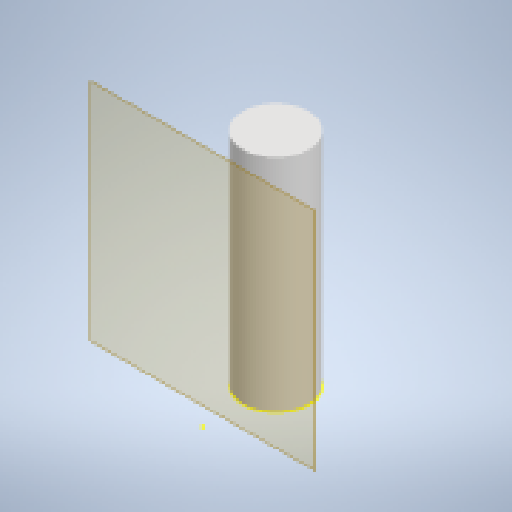
# Autodesk Inventor part: 21700
Saved by Autodesk Inventor 2024.2 (Build 282272000, 272)
## iProperties
Created: 2025-10-05
Part Number: 21700
Material: Типовые
Document SubType Name: Modeling
Designer: katya_notebook
Density: 1 g/cm^3
Appearance: По умолчанию
Author: katya_notebook
Autodesk Inventor part; units mm, degrees
ref_plane "YZ Plane" through (0, 0, 0) normal (1, 0, 0) x (0, 1, 0)
ref_plane "XZ Plane" through (0, 0, 0) normal (0, 1, 0) x (-1, 0, 0)
ref_plane "XY Plane" through (0, 0, 0) normal (0, 0, 1) x (1, 0, 0)
sketch "Эскиз1" plane through (0, 0, 0) normal (0, 1, 0) x (-1, 0, 0)
  circle A0 centre (0, 0) radius 10.5
  dimension "d0" = 21
  constraints: 1 centre point, 1 coincident
  measures "d0" diameter of A0
extrude "Выдавливание1" add sketch "Эскиз1" along normal blind 70
sketch "Эскиз2" plane through (0, 0, 0) normal (0, -1, 0) x (1, 0, 0)
  circle A0 centre (0, 0) radius 10.5 projected
  line L0 (-10.5, 0) -> (10.5, 0)
  line L1 (0, 10.5) -> (0, -10.5)
  constraints: 4 end point, 4 point on circle, 1 coincident, 1 horizontal, 1 perpendicular
ref_plane "РабПлоскость1" through (0, 41.5126, 23.0718) normal (0, 0, 1) x (0, 1, 0)
sketch "Эскиз3" plane through (0, 41.5126, 23.0718) normal (0, 0, 1) x (0, 1, 0)
  point P0 (-41.5126, 0)
